Autodesk Fusion 360 part; units mm, degrees
note: some values were not read from the file. Set by a fixed rule: which sketch regions a step uses.
(part 2 of 3)
  arc A260 (-243, 45) -> (-241, 43) centre (-241, 45) ccw
  line L698 (-243, 45) -> (-243, 51)
  arc A261 (-243, 51) -> (-245, 53) centre (-245, 51) ccw
  line L699 (-245, 53) -> (-267, 53)
  line L700 (-267, 124) -> (-204, 124.0001)
  arc A262 (-204, 124.0001) -> (-202, 126.0001) centre (-204, 126.0001) ccw
  line L701 (-202, 126.0001) -> (-202, 135)
  line L702 (-202, 135) -> (-197, 135)
  line L703 (-197, 135) -> (-197, 133.0001)
  arc A263 (-197, 133.0001) -> (-195, 131.0001) centre (-195, 133.0001) ccw
  arc A264 (-172, 127) -> (-176, 131.0001) centre (-176, 127.0001) ccw
  line L704 (-172, 123) -> (-172, 127)
  arc A265 (-176, 119.0001) -> (-172, 123) centre (-176, 123.0001) ccw
  arc A266 (-195, 119) -> (-197, 117) centre (-195, 117) ccw
  line L705 (-197, 117) -> (-197, 115)
  line L706 (-197, 115) -> (-200, 115)
  arc A267 (-200, 115) -> (-202, 113) centre (-200, 113) ccw
  line L707 (-202, 109) -> (-202, 113)
  arc A268 (-204, 107) -> (-202, 109) centre (-204, 109) ccw
  line L708 (-204, 107) -> (-241, 107)
  arc A269 (-241, 107) -> (-243, 105) centre (-241, 105) ccw
  line L709 (-243, 105) -> (-243, 99)
  arc A270 (-245, 97) -> (-243, 99) centre (-245, 99) ccw
  line L710 (-245, 97) -> (-267, 97)
  arc A271 (-332, 126.0001) -> (-330, 124.0001) centre (-330, 126.0001) ccw
  line L711 (-332, 126.0001) -> (-332, 135)
  line L712 (-332, 135) -> (-337, 135)
  line L713 (-337, 135) -> (-337, 133.0001)
  arc A272 (-339, 131.0001) -> (-337, 133.0001) centre (-339, 133.0001) ccw
  arc A273 (-358, 131.0001) -> (-362, 127) centre (-358, 127.0001) ccw
  line L714 (-362, 123) -> (-362, 127)
  arc A274 (-362, 123) -> (-358, 119.0001) centre (-358, 123.0001) ccw
  arc A275 (-337, 117) -> (-339, 119) centre (-339, 117) ccw
  line L715 (-337, 117) -> (-337, 115)
  line L716 (-337, 115) -> (-334, 115)
  arc A276 (-332, 113) -> (-334, 115) centre (-334, 113) ccw
  line L717 (-332, 109) -> (-332, 113)
  arc A277 (-332, 109) -> (-330, 107) centre (-330, 109) ccw
  line L718 (-330, 107) -> (-287, 107)
  arc A278 (-285, 105) -> (-287, 107) centre (-287, 105) ccw
  line L719 (-285, 105) -> (-285, 99)
  arc A279 (-285, 99) -> (-283, 97) centre (-283, 99) ccw
  line L720 (-283, 97) -> (-267, 97)
  line L721 (-267, 124) -> (-330, 124.0001)
  line L722 (-327, 5) -> (-327, 10)
  line L723 (-327, 10) -> (-307, 10)
  arc A280 (-223, 3) -> (-225, 5) centre (-225, 3) ccw
  line L724 (-225, 5) -> (-227, 5)
  line L725 (-227, 5) -> (-227, 10)
  line L726 (-207, 10) -> (-227, 10)
  line L727 (-207, 5) -> (-207, 10)
  line L728 (-207, 5) -> (-209.0021, 5)
  arc A281 (-209.0021, 5) -> (-211.0021, 2.9998) centre (-209.0021, 3) ccw
  line L729 (-211, -15.9146) -> (-211.0021, 2.9998)
  arc A282 (-215, -19.9102) -> (-211, -15.9146) centre (-215, -15.9102) ccw
  line L730 (-219, -19.9102) -> (-215, -19.9102)
  arc A283 (-223, -15.9116) -> (-219, -19.9102) centre (-219, -15.9102) ccw
  line L731 (-223, -15.9116) -> (-223, 3)
  line L732 (-225, 145) -> (-227, 145)
  line L733 (-227, 145) -> (-227, 140)
  line L734 (-207, 140) -> (-227, 140)
  line L735 (-207, 145) -> (-207, 140)
  line L736 (-207, 145) -> (-209.0021, 145)
  arc A284 (-211.0021, 147.0002) -> (-209.0021, 145) centre (-209.0021, 147) ccw
  line L737 (-211.0007, 166.0733) -> (-211.0021, 147.0002)
  arc A285 (-211.0007, 166.0733) -> (-215, 170) centre (-215, 166) ccw
  line L738 (-219, 170) -> (-215, 170)
  arc A286 (-219, 170) -> (-223, 166.0009) centre (-219, 166) ccw
  line L739 (-223, 166.0009) -> (-223, 147)
  arc A287 (-225, 145) -> (-223, 147) centre (-225, 147) ccw
  arc A288 (-311, 147) -> (-309, 145) centre (-309, 147) ccw
  line L740 (-309, 145) -> (-307, 145)
  line L741 (-307, 145) -> (-307, 140)
  line L742 (-327, 140) -> (-307, 140)
  line L743 (-327, 145) -> (-327, 140)
  line L744 (-327, 145) -> (-324.9979, 145)
  arc A289 (-324.9979, 145) -> (-322.9979, 147.0002) centre (-324.9979, 147) ccw
  line L745 (-322.9993, 165.9261) -> (-322.9979, 147.0002)
  arc A290 (-319, 170) -> (-322.9993, 165.9261) centre (-319, 166) ccw
  line L746 (-315, 170) -> (-319, 170)
  arc A291 (-311, 166.0009) -> (-315, 170) centre (-315, 166) ccw
  line L747 (-311, 166.0009) -> (-311, 147)
  circle A292 centre (43.5, 122.75) radius 3
  circle A293 centre (58.5, 122.75) radius 3
  circle A294 centre (73.5, 122.75) radius 3
  circle A295 centre (73.5, 27.25) radius 3
  arc A296 (79.466, 30.6504) -> (82, 35) centre (77, 35) ccw
  circle A297 centre (43.5, 17.25) radius 2.5
  circle A298 centre (58.5, 17.25) radius 2.5
  circle A299 centre (73.5, 132.75) radius 2.5
  circle A300 centre (58.5, 132.75) radius 2.5
  circle A301 centre (43.5, 132.75) radius 2.5
  line L748 (35, 5) -> (35, 10)
  line L749 (57.5, 5) -> (35, 5)
  line L750 (57.5, 10) -> (35, 10)
  line L751 (57.5, 5) -> (80, 5)
  line L752 (80, 5) -> (80, 10)
  line L753 (80, 10) -> (57.5, 10)
  line L754 (-10, -124) -> (-10, -114)
  line L755 (-10, -59) -> (-10, -69)
  line L756 (-13, -74) -> (-12, -74)
  line L757 (-12, -109) -> (-13, -109)
  line L758 (-15, -117) -> (-15, -114)
  arc A302 (-13, -109) -> (-14.3301, -109.5064) centre (-13, -111) ccw
  arc A303 (-12, -109) -> (-10, -107) centre (-12, -107) ccw
  arc A304 (-10, -76) -> (-12, -74) centre (-12, -76) ccw
  line L759 (-10, -76) -> (-10, -80.6987)
  line L760 (-10, -88.0192) -> (-10, -98.0192)
  arc A305 (-15, -72) -> (-14.9997, -72.0383) centre (-13, -72) ccw
  arc A306 (-14.3301, -73.4936) -> (-13, -74) centre (-13, -72) ccw
  line L761 (-15, -72) -> (-15, -67)
  line L762 (-135.6699, -107.8397) -> (-140, -105.3397)
  line L763 (-135.6699, -109.5064) -> (-135.6699, -107.8397)
  arc A307 (-135.6699, -109.5064) -> (-137, -109) centre (-137, -111) ccw
  line L764 (-138, -109) -> (-137, -109)
  line L765 (-140, -105.3398) -> (-140, -107)
  arc A308 (-140, -107) -> (-138, -109) centre (-138, -107) ccw
  line L766 (-139.9897, -75.7973) -> (-140, -80.6987)
  line L767 (-140, -80.6987) -> (-135.6699, -78.1987)
  arc A309 (-137, -74) -> (-135.6699, -73.4936) centre (-137, -72) ccw
  line L768 (-137, -74) -> (-138, -74)
  arc A310 (-138, -74) -> (-140, -76) centre (-138, -76) ccw
  line L769 (-140, -76) -> (-140, -80.6987)
  line L770 (-135.6699, -78.1987) -> (-135.6699, -73.4936)
  arc A311 (-133, -64) -> (-135, -66) centre (-133, -66) ccw
  line L771 (-133, -64) -> (-132, -64)
  arc A312 (-132, -64) -> (-131.6546, -63.9699) centre (-132, -62) ccw
  line L772 (-130.6699, -64.5385) -> (-131.6546, -63.9699)
  line L773 (-130.6699, -69.5385) -> (-130.6699, -64.5385)
  line L774 (-135, -72.0385) -> (-130.6699, -69.5385)
  line L775 (-135.0004, -72.0383) -> (-135, -72.0385)
  arc A313 (-135.0004, -72.0383) -> (-135, -72) centre (-137, -72) ccw
  line L776 (-135, -67) -> (-135, -66)
  line L777 (-135, -72) -> (-135, -67)
  line L778 (-90, -124) -> (-90, -129)
  line L779 (-90, -124) -> (-115, -124)
  line L780 (-115, -124) -> (-115, -129)
  line L781 (-115, -129) -> (-135, -129)
  line L782 (-135, -124) -> (-140, -124)
  line L783 (-140, -124) -> (-140, -114)
  line L784 (-145, -114) -> (-140, -114)
  line L785 (-145, -69) -> (-145, -114)
  line L786 (-140, -69) -> (-145, -69)
  line L787 (-140, -59) -> (-140, -69)
  line L788 (-140, -59) -> (-135, -59)
  line L789 (-135, -54) -> (-135, -59)
  line L790 (-135, -49) -> (-135, -54)
  arc A314 (-131.8566, -44.3575) -> (-135, -49) centre (-130, -49) ccw
  arc A315 (-115, -49) -> (-118.1434, -44.3575) centre (-120, -49) ccw
  line L791 (-115, -54) -> (-115, -49)
  line L792 (-115, -59) -> (-115, -54)
  line L793 (-115, -59) -> (-94.5, -59)
  line L794 (-94.5, -59) -> (-94.5, -39)
  arc A316 (-89.5, -34) -> (-94.5, -39) centre (-89.5, -39) ccw
  line L795 (-135, -129) -> (-135, -124)
  line L796 (-90, -129) -> (-60, -129)
  circle A317 centre (-85, -48) radius 4.075
  circle A318 centre (-371, 85) radius 4.075
  line L797 (-438, 19) -> (-442, 19)
  line L798 (-444, 17) -> (-444, 15.5)
  line L799 (-442, 13.5) -> (-438, 13.5)
  line L800 (-436, 15.5) -> (-436, 17)
  arc A319 (-436, 17) -> (-438, 19) centre (-438, 17) ccw
  arc A320 (-438, 13.5) -> (-436, 15.5) centre (-438, 15.5) ccw
  arc A321 (-444, 15.5) -> (-442, 13.5) centre (-442, 15.5) ccw
  arc A322 (-442, 19) -> (-444, 17) centre (-442, 17) ccw
  arc A323 (-438, 131) -> (-436, 133) centre (-438, 133) ccw
  line L801 (-438, 131) -> (-442, 131)
  arc A324 (-444, 133) -> (-442, 131) centre (-442, 133) ccw
  line L802 (-444, 133) -> (-444, 134.5)
  arc A325 (-442, 136.5) -> (-444, 134.5) centre (-442, 134.5) ccw
  line L803 (-442, 136.5) -> (-438, 136.5)
  arc A326 (-436, 134.5) -> (-438, 136.5) centre (-438, 134.5) ccw
  line L804 (-436, 134.5) -> (-436, 133)
  arc A327 (41.7475, 118.6053) -> (45.2525, 118.6053) centre (43.5, 122.75) ccw
  line L805 (34, 119) -> (39.8003, 119)
  line L806 (47.1997, 119) -> (54.8003, 119)
  arc A328 (56.7475, 118.6053) -> (60.2525, 118.6053) centre (58.5, 122.75) ccw
  line L807 (62.1997, 119) -> (69.8003, 119)
  line L808 (77.1997, 119) -> (81, 119)
  arc A329 (71.7475, 118.6053) -> (75.2525, 118.6053) centre (73.5, 122.75) ccw
  arc A330 (41.7475, 118.6053) -> (39.8003, 119) centre (39.8003, 114) ccw
  arc A331 (47.1997, 119) -> (45.2525, 118.6053) centre (47.1997, 114) ccw
  arc A332 (56.7475, 118.6053) -> (54.8003, 119) centre (54.8003, 114) ccw
  arc A333 (62.1997, 119) -> (60.2525, 118.6053) centre (62.1997, 114) ccw
  arc A334 (71.7475, 118.6053) -> (69.8003, 119) centre (69.8003, 114) ccw
  arc A335 (77.1997, 119) -> (75.2525, 118.6053) centre (77.1997, 114) ccw
  line L809 (-82.0096, -106.5) -> (-77.9904, -106.5)
  line L810 (-72.0096, -106.5) -> (-67.9904, -106.5)
  arc A336 (-289.5, 21) -> (-291.5, 23) centre (-291.5, 21) ccw
  line L811 (-291.5, 23) -> (-327, 23)
  arc A337 (-327, 23) -> (-329, 21) centre (-327, 21) ccw
  line L812 (-329, 15) -> (-329, 21)
  arc A338 (-329, 15) -> (-327, 13) centre (-327, 15) ccw
  line L813 (-249.5, 23) -> (-284.5, 23)
  arc A339 (-284.5, 23) -> (-286.5, 21) centre (-284.5, 21) ccw
  arc A340 (-247.5, 21) -> (-249.5, 23) centre (-249.5, 21) ccw
  line L814 (-337, 108) -> (-337, 92.5)
  arc A341 (-337, 108) -> (-339, 110) centre (-339, 108) ccw
  line L815 (-339, 110) -> (-340, 110)
  arc A342 (-342, 112) -> (-340, 110) centre (-340, 112) ccw
  line L816 (-342, 112) -> (-342, 112.9999)
  arc A343 (-342, 112.9999) -> (-344, 114.9999) centre (-344, 112.9999) ccw
  arc A344 (-366, 122.9999) -> (-358, 114.9999) centre (-358, 122.9999) ccw
  line L817 (-366, 126.9998) -> (-366, 122.9999)
  arc A345 (-358, 134.9998) -> (-366, 126.9998) centre (-358, 126.9998) ccw
  arc A346 (-344, 134.9999) -> (-342, 136.9999) centre (-344, 136.9999) ccw
  line L818 (-342, 136.9999) -> (-342.0001, 145)
  arc A347 (-337, 150) -> (-342.0001, 145) centre (-337, 145) ccw
  line L819 (-337, 150) -> (-329, 150)
  arc A348 (-329, 150) -> (-327, 152) centre (-329, 152) ccw
  line L820 (-327, 166) -> (-327, 152)
  arc A349 (-319, 174) -> (-327, 166) centre (-319, 166) ccw
  line L821 (-315, 174) -> (-319, 174)
  arc A350 (-307, 166.0013) -> (-315, 174) centre (-315, 166) ccw
  line L822 (-307, 152) -> (-307, 166.0013)
  arc A351 (-307, 152) -> (-305, 150) centre (-305, 152) ccw
  line L823 (-305, 150) -> (-304, 150)
  arc A352 (-302, 148) -> (-304, 150) centre (-304, 148) ccw
  line L824 (-302, 147) -> (-302, 148)
  arc A353 (-302, 147) -> (-300, 145) centre (-300, 147) ccw
  line L825 (-300, 145) -> (-286.5, 145)
  line L826 (-247.5, 144.9999) -> (-233.9999, 144.9999)
  arc A354 (-233.9999, 144.9999) -> (-231.9997, 147.0001) centre (-233.9999, 147.0001) ccw
  line L827 (-231.9997, 147.0001) -> (-231.9997, 147.9994)
  arc A355 (-229.999, 150.0001) -> (-231.9997, 147.9994) centre (-229.999, 147.9994) ccw
  line L828 (-229, 150.0001) -> (-229.999, 150.0001)
  arc A356 (-229, 150.0001) -> (-227, 152.0001) centre (-229, 152.0001) ccw
  line L829 (-227, 152.0001) -> (-227, 166.002)
  arc A357 (-219, 174) -> (-227, 166.002) centre (-219, 166) ccw
  line L830 (-219, 174) -> (-215, 174)
  arc A358 (-207, 166) -> (-215, 174) centre (-215, 166) ccw
  line L831 (-207, 166) -> (-207, 152.0001)
  arc A359 (-207, 152.0001) -> (-205, 150.0001) centre (-205, 152.0001) ccw
  line L832 (-197, 150.0001) -> (-205, 150.0001)
  arc A360 (-192, 145.0001) -> (-197, 150.0001) centre (-197, 145.0001) ccw
  line L833 (-192, 145.0001) -> (-192, 136.9999)
  arc A361 (-192, 136.9999) -> (-190, 134.9999) centre (-190, 136.9999) ccw
  arc A362 (-168, 126.9998) -> (-175.9914, 134.9998) centre (-176, 126.9998) ccw
  line L834 (-168, 126.9998) -> (-168, 122.9999)
  arc A363 (-176, 114.9999) -> (-168, 122.9999) centre (-176, 122.9999) ccw
  arc A364 (-190, 114.9999) -> (-192, 112.9999) centre (-190, 112.9999) ccw
  line L835 (-192, 112) -> (-192, 112.9999)
  arc A365 (-194, 110) -> (-192, 112) centre (-194, 112) ccw
  line L836 (-195, 110) -> (-194, 110)
  arc A366 (-195, 110) -> (-197, 108) centre (-195, 108) ccw
  line L837 (-197, 108) -> (-197, 90)
  line L838 (-197, 90) -> (-202, 90)
  line L839 (-202, 90) -> (-202, 75)
  arc A367 (-406.5714, 84.2084) -> (-403.2084, 87.5714) centre (-408, 89) ccw
  arc A368 (-401.2918, 89) -> (-403.2084, 87.5714) centre (-401.2918, 87) ccw
  arc A369 (-386.7082, 61) -> (-384.7916, 62.4286) centre (-386.7082, 63) ccw
  arc A370 (-381.4286, 65.7916) -> (-384.7916, 62.4286) centre (-380, 61) ccw
  arc A371 (-381.4286, 65.7916) -> (-380, 67.7082) centre (-382, 67.7082) ccw
  arc A372 (-406.5714, 84.2084) -> (-408, 82.2918) centre (-406, 82.2918) ccw
  circle A373 centre (-408, 89) radius 1
  circle A374 centre (-380, 61) radius 1
  line L840 (-408, 82.2918) -> (-408, 67.7082)
  line L841 (-401.2918, 61) -> (-386.7082, 61)
  line L842 (-401.2918, 89) -> (-386.7082, 89)
  line L843 (-380, 82.2918) -> (-380, 67.7082)
  line L844 (-104, 5) -> (-86, 5)
  line L845 (-56, 5) -> (-38, 5)
  line L846 (-104, 145) -> (-86, 145)
  line L847 (-56, 145) -> (-38, 145)
  line L848 (-141, 90) -> (-141, 108)
  line L849 (-141, 60) -> (-141, 42)
  line L850 (-302, 8) -> (-291.5, 8)
  line L851 (-327, 13) -> (-306, 13)
  line L852 (-304, 11) -> (-304, 10)
  line L853 (-289.5, 21) -> (-289.5, 10)
  arc A375 (-304, 11) -> (-306, 13) centre (-306, 11) ccw
  arc A376 (-304, 10) -> (-302, 8) centre (-302, 10) ccw
  arc A377 (-291.5, 8) -> (-289.5, 10) centre (-291.5, 10) ccw
  arc A378 (-244.5001, 10) -> (-242.5001, 8) centre (-242.5001, 10) ccw
  line L854 (-232.0001, 7.9999) -> (-242.5001, 8)
  arc A379 (-232.0001, 7.9999) -> (-230.0001, 9.9999) centre (-232.0001, 9.9999) ccw
  line L855 (-230.0001, 10.9999) -> (-230.0001, 9.9999)
  arc A380 (-228.0001, 12.9999) -> (-230.0001, 10.9999) centre (-228.0001, 10.9999) ccw
  line L856 (-207.0001, 12.9999) -> (-228.0001, 12.9999)
  arc A381 (-207.0001, 12.9999) -> (-205.0001, 14.9999) centre (-207.0001, 14.9999) ccw
  line L857 (-205.0001, 14.9999) -> (-205.0001, 20.9999)
  arc A382 (-205.0001, 20.9999) -> (-207.0001, 22.9999) centre (-207.0001, 20.9999) ccw
  line L858 (-242.4962, 23) -> (-207.0001, 22.9999)
  arc A383 (-242.4962, 23) -> (-244.5001, 21) centre (-242.5001, 21) ccw
  line L859 (-244.5001, 21) -> (-244.5001, 10)
  line L860 (-329, 135) -> (-329, 129)
  arc A384 (-327, 137) -> (-329, 135) centre (-327, 135) ccw
  line L861 (-327, 137) -> (-306, 137)
  arc A385 (-306, 137) -> (-304, 139) centre (-306, 139) ccw
  line L862 (-304, 139) -> (-304, 140)
  arc A386 (-302, 142) -> (-304, 140) centre (-302, 140) ccw
  line L863 (-302, 142) -> (-291.5, 142)
  arc A387 (-289.5, 140) -> (-291.5, 142) centre (-291.5, 140) ccw
  line L864 (-289.5, 129) -> (-289.5, 140)
  arc A388 (-291.5, 127) -> (-289.5, 129) centre (-291.5, 129) ccw
  line L865 (-291.5, 127) -> (-327, 127)
  arc A389 (-329, 129) -> (-327, 127) centre (-327, 129) ccw
  arc A390 (-207.0001, 127.0001) -> (-205.0001, 129.0001) centre (-207.0001, 129.0001) ccw
  line L866 (-205.0001, 135.0001) -> (-205.0001, 129.0001)
  arc A391 (-205.0001, 135.0001) -> (-207.0001, 137.0001) centre (-207.0001, 135.0001) ccw
  line L867 (-207.0001, 137.0001) -> (-228.0001, 137.0001)
  arc A392 (-230.0001, 139.0001) -> (-228.0001, 137.0001) centre (-228.0001, 139.0001) ccw
  line L868 (-230.0001, 139.0001) -> (-230.0001, 140.0001)
  arc A393 (-230.0001, 140.0001) -> (-232.0001, 142.0001) centre (-232.0001, 140.0001) ccw
  line L869 (-232.0001, 142.0001) -> (-242.5001, 142)
  arc A394 (-242.5001, 142) -> (-244.5001, 140) centre (-242.5001, 140) ccw
  line L870 (-244.5001, 129) -> (-244.5001, 140)
  arc A395 (-244.5001, 129) -> (-242.4962, 127) centre (-242.5001, 129) ccw
  line L871 (-242.4962, 127) -> (-207.0001, 127.0001)
  line L872 (-437, 10) -> (-392, 10)
  line L873 (-414.5, 145) -> (-392, 145)
  line L874 (-414.5, 145) -> (-437, 145)
  line L875 (-437, 145) -> (-437, 140)
  line L876 (-437, 140) -> (-392, 140)
  line L877 (-392, 145) -> (-392, 140)
  line L878 (-418.1847, 13) -> (-405.8153, 13)
  arc A396 (-422.7659, 14.1111) -> (-418.1847, 13) centre (-418.1847, 23) ccw
  arc A397 (-405.8153, 13) -> (-401.2341, 14.1111) centre (-405.8153, 23) ccw
  line L879 (-136, 10) -> (-141, 10)
  line L880 (-141, 5) -> (-136, 5)
  line L881 (-136, 5) -> (-136, 10)
  line L882 (-141, 10) -> (-141, 5)
  line L883 (-1, 5) -> (-6, 5)
  line L884 (-6, 5) -> (-6, 10)
  line L885 (-6, 10) -> (-1, 10)
  line L886 (-1, 10) -> (-1, 5)
  line L887 (-136, 145) -> (-136, 140)
  line L888 (-136, 140) -> (-141, 140)
  line L889 (-141, 140) -> (-141, 145)
  line L890 (-141, 145) -> (-136, 145)
  line L891 (-6, 145) -> (-6, 140)
  line L892 (-6, 140) -> (-1, 140)
  line L893 (-1, 140) -> (-1, 145)
  line L894 (-1, 145) -> (-6, 145)
  arc A398 (-403.2084, 62.4286) -> (-406.5714, 65.7916) centre (-408, 61) ccw
  arc A399 (-411.2142, 57.17) -> (-406.0857, 56.381) centre (-408, 61) ccw
  arc A400 (-401.2341, 14.1111) -> (-402.0555, 56.2922) centre (-412, 35) ccw
  arc A401 (-415.0846, 58.2967) -> (-422.7659, 14.1111) centre (-412, 35) ccw
  arc A402 (-411.2142, 57.17) -> (-415.0846, 58.2967) centre (-414.4283, 53.3399) ccw
  arc A403 (-402.0555, 56.2922) -> (-406.0857, 56.381) centre (-404.1714, 51.7619) ccw
  line L895 (-418.1847, 137) -> (-405.8153, 137)
  arc A404 (-401.2341, 135.8889) -> (-405.8153, 137) centre (-405.8153, 127) ccw
  arc A405 (-402.0555, 93.7078) -> (-401.2341, 135.8889) centre (-412, 115) ccw
  arc A406 (-406.0857, 93.619) -> (-402.0555, 93.7078) centre (-404.1714, 98.2381) ccw
  arc A407 (-406.0857, 93.619) -> (-411.2142, 92.83) centre (-408, 89) ccw
  arc A408 (-415.0846, 91.7033) -> (-411.2142, 92.83) centre (-414.4283, 96.6601) ccw
  arc A409 (-422.7659, 135.8889) -> (-415.0846, 91.7033) centre (-412, 115) ccw
  arc A410 (-418.1847, 137) -> (-422.7659, 135.8889) centre (-418.1847, 127) ccw
  circle A411 centre (-125, -40) radius 2.5
  arc A412 (-119.3006, -41.8753) -> (-130.6994, -41.8753) centre (-125, -40) ccw
  arc A413 (-119.3006, -41.8753) -> (-118.1434, -44.3575) centre (-117.4008, -42.5004) ccw
  arc A414 (-131.8566, -44.3575) -> (-130.6994, -41.8753) centre (-132.5992, -42.5004) ccw
  arc A415 (-15, -49) -> (-18.1435, -44.3575) centre (-20, -49) ccw
  arc A416 (-19.3006, -41.8753) -> (-18.1435, -44.3575) centre (-17.4008, -42.5004) ccw
  arc A417 (-19.3006, -41.8753) -> (-30.6994, -41.8753) centre (-25, -40) ccw
  circle A418 centre (-25, -40) radius 2.5
  arc A419 (-31.8566, -44.3575) -> (-35, -49) centre (-30, -49) ccw
  arc A420 (-31.8566, -44.3575) -> (-30.6994, -41.8753) centre (-32.5992, -42.5004) ccw
  line L896 (-286.5, 5) -> (-286.5, 11)
  line L897 (-284.5, 13) -> (-249.5, 13)
  line L898 (-247.5, 11) -> (-247.5, 5.0001)
  arc A421 (-249.5, 16) -> (-247.5, 18) centre (-249.5, 18) ccw
  line L899 (-249.5, 16) -> (-284.5, 16)
  arc A422 (-286.5, 18) -> (-284.5, 16) centre (-284.5, 18) ccw
  arc A423 (-284.5, 13) -> (-286.5, 11) centre (-284.5, 11) ccw
  arc A424 (-247.5, 11) -> (-249.5, 13) centre (-249.5, 11) ccw
  line L900 (-286.5, 18) -> (-286.5, 21)
  line L901 (-247.5, 21) -> (-247.5, 18)
  line L902 (-284.5, 137) -> (-249.5, 137)
  arc A425 (-284.5, 134) -> (-286.5, 132) centre (-284.5, 132) ccw
  line L903 (-286.5, 132) -> (-286.5, 129)
  arc A426 (-286.5, 129) -> (-284.5, 127) centre (-284.5, 129) ccw
  line L904 (-249.5, 127) -> (-284.5, 127)
  arc A427 (-249.5, 127) -> (-247.5, 129) centre (-249.5, 129) ccw
  line L905 (-247.5, 129) -> (-247.5, 132)
  arc A428 (-247.5, 132) -> (-249.5, 134) centre (-249.5, 132) ccw
  line L906 (-249.5, 134) -> (-284.5, 134)
  arc A429 (-286.5, 139) -> (-284.5, 137) centre (-284.5, 139) ccw
  line L907 (-286.5, 145) -> (-286.5, 139)
  line L908 (-247.5, 139) -> (-247.5, 144.9999)
  arc A430 (-249.5, 137) -> (-247.5, 139) centre (-249.5, 139) ccw
  line L909 (-337, 92.5) -> (-331, 92.5)
  line L910 (-337, 57.5) -> (-331, 57.5)
  line L911 (-329, 90.5) -> (-329, 59.5)
  arc A431 (-329, 90.5) -> (-331, 92.5) centre (-331, 90.5) ccw
  arc A432 (-331, 57.5) -> (-329, 59.5) centre (-331, 59.5) ccw
  arc A433 (76.1918, 30.8561) -> (70.8974, 30.9211) centre (73.5, 27.25) ccw
  line L912 (38, 30) -> (68.0057, 30)
  arc A434 (68.0057, 30) -> (70.8974, 30.9211) centre (68.0057, 35) ccw
  arc A435 (76.1918, 30.8561) -> (79.466, 30.6504) centre (77.9864, 33.2602) ccw
  line L913 (-195, 18.9999) -> (-176, 18.9999)
  line L914 (-190, 15.0001) -> (-175.9914, 15.0002)
  line L915 (-190, 35.0001) -> (-176, 35.0001)
  line L916 (-195, 31) -> (-176, 30.9999)
  line L917 (-195, 119) -> (-176, 119.0001)
  line L918 (-190, 114.9999) -> (-176, 114.9999)
  line L919 (-195, 131.0001) -> (-176, 131.0001)
  line L920 (-190, 134.9999) -> (-175.9914, 134.9998)
  line L921 (-358, 134.9998) -> (-344, 134.9999)
  line L922 (-358, 131.0001) -> (-339, 131.0001)
  line L923 (-358, 119.0001) -> (-339, 119)
  line L924 (-358, 114.9999) -> (-344, 114.9999)
  line L925 (-358, 35.0001) -> (-344, 35.0001)
  line L926 (-358, 30.9999) -> (-339, 31)
  line L927 (-358, 18.9999) -> (-339, 18.9999)
  line L928 (-358, 15.0002) -> (-344, 15.0001)
  circle A436 centre (-240, 91) radius 1.5
  circle A437 centre (-208, 91) radius 1.5
  circle A438 centre (-240, 59) radius 1.5
  circle A439 centre (-208, 59) radius 1.5
  line L929 (-240, 65.3246) -> (-240, 84.6754)
  line L930 (-214.3246, 59) -> (-233.6754, 59)
  line L931 (-238.5, 59) -> (-240, 59)
  arc A440 (-236.386, 60.7143) -> (-238.2857, 62.614) centre (-240, 59) ccw
  arc A441 (-238.2857, 87.386) -> (-236.386, 89.2857) centre (-240, 91) ccw
  arc A442 (-211.614, 89.2857) -> (-209.7143, 87.386) centre (-208, 91) ccw
  line L932 (-233.6754, 91) -> (-214.3246, 91)
  line L933 (-208, 84.6754) -> (-208, 65.3246)
  arc A443 (-209.7143, 62.614) -> (-211.614, 60.7143) centre (-208, 59) ccw
  arc A444 (-238.2857, 87.386) -> (-240, 84.6754) centre (-237, 84.6754) ccw
  arc A445 (-233.6754, 91) -> (-236.386, 89.2857) centre (-233.6754, 88) ccw
  arc A446 (-240, 65.3246) -> (-238.2857, 62.614) centre (-237, 65.3246) ccw
  arc A447 (-236.386, 60.7143) -> (-233.6754, 59) centre (-233.6754, 62) ccw
  arc A448 (-214.3246, 59) -> (-211.614, 60.7143) centre (-214.3246, 62) ccw
  arc A449 (-209.7143, 62.614) -> (-208, 65.3246) centre (-211, 65.3246) ccw
  arc A450 (-208, 84.6754) -> (-209.7143, 87.386) centre (-211, 84.6754) ccw
  arc A451 (-211.614, 89.2857) -> (-214.3246, 91) centre (-214.3246, 88) ccw
  circle A452 centre (30, -80) radius 1
  circle A453 centre (30, -108) radius 1
  arc A454 (31.1111, -82.2395) -> (32.2395, -81.1111) centre (30, -80) ccw
  line L934 (30, -103.9689) -> (30, -84.0311)
  line L935 (34.0311, -80) -> (44, -80)
  arc A455 (30, -103.9689) -> (31.1111, -105.7605) centre (32, -103.9689) ccw
  arc A456 (34.0311, -80) -> (32.2395, -81.1111) centre (34.0311, -82) ccw
  arc A457 (31.1111, -82.2395) -> (30, -84.0311) centre (32, -84.0311) ccw
  line L936 (19.75, -89.25) -> (19.75, -95.75)
  line L937 (22.25, -89.2502) -> (22.25, -95.75)
  arc A458 (22.25, -89.2502) -> (19.75, -89.25) centre (21, -89.25) ccw
  arc A459 (19.75, -95.75) -> (22.25, -95.75) centre (21, -95.75) ccw
  line L938 (-75, -55) -> (-90, -55)
  line L939 (-92, -57) -> (-92, -103)
  line L940 (-90, -105) -> (-60, -105)
  line L941 (-58, -103) -> (-58, -57)
  line L942 (-60, -55) -> (-75, -55)
  arc A460 (22.25, -107.25) -> (19.75, -107.25) centre (21, -107.25) ccw
  line L943 (19.75, -113.75) -> (19.75, -107.25)
  arc A461 (19.75, -113.75) -> (22.25, -113.7498) centre (21, -113.75) ccw
  line L944 (22.25, -113.7498) -> (22.25, -107.25)
  line L945 (-87.9002, -106.5521) -> (-92.1651, -106.5898)
  line L946 (-62.0096, -106.5) -> (-57.9904, -106.5)
  arc A462 (-90, -55) -> (-92, -57) centre (-90, -57) ccw
  arc A463 (-58, -57) -> (-60, -55) centre (-60, -57) ccw
  arc A464 (-60, -105) -> (-58, -103) centre (-60, -103) ccw
  arc A465 (-92, -103) -> (-90, -105) centre (-90, -103) ccw
  line L947 (-89.5, -34) -> (-60.5, -34)
  arc A466 (32.5, -108) -> (31.1111, -105.7605) centre (30, -108) ccw
  line L948 (21, -99.7811) -> (21, -103.2189)
  line L949 (32.5, -108) -> (32.5, -110.7498)
  line L950 (29.5, -113.7498) -> (25.0312, -113.7498)
  line L951 (18.5, -113.7498) -> (18.5, -107.25)
  line L952 (18.5, -95.75) -> (18.5, -89.25)
  arc A467 (18.5, -113.7498) -> (23.2396, -114.861) centre (21, -113.75) ccw
  arc A468 (19.8889, -105.0105) -> (18.5, -107.25) centre (21, -107.25) ccw
  arc A469 (18.5, -95.75) -> (19.8889, -97.9895) centre (21, -95.75) ccw
  line L953 (30, -77.5) -> (44, -77.5)
  arc A470 (31.1111, -82.2395) -> (32.2395, -81.1111) centre (30, -80) ccw
  arc A471 (30, -77.5) -> (27.5, -80) centre (30, -80) ccw
  arc A472 (21, -99.7811) -> (19.8889, -97.9895) centre (19, -99.7811) ccw
  arc A473 (19.8889, -105.0105) -> (21, -103.2189) centre (19, -103.2189) ccw
  arc A474 (25.0312, -113.7498) -> (23.2396, -114.861) centre (25.0312, -115.7498) ccw
  arc A475 (29.5, -113.7498) -> (32.5, -110.7498) centre (29.5, -110.7498) ccw
  circle A476 centre (58, -108) radius 1
  line L954 (68.25, -113.75) -> (68.25, -107.25)
  arc A477 (65.75, -113.7498) -> (68.25, -113.75) centre (67, -113.75) ccw
  arc A478 (68.25, -107.25) -> (65.75, -107.25) centre (67, -107.25) ccw
  line L955 (65.75, -113.7498) -> (65.75, -107.25)
  arc A479 (65.75, -95.75) -> (68.25, -95.75) centre (67, -95.75) ccw
  line L956 (68.25, -89.25) -> (68.25, -95.75)
  arc A480 (68.25, -89.25) -> (65.75, -89.2502) centre (67, -89.25) ccw
  line L957 (65.75, -89.2502) -> (65.75, -95.75)
  circle A481 centre (58, -80) radius 1
  line L958 (-55.25, -93.75) -> (-48.75, -93.75)
  line L959 (-55.25, -96.25) -> (-48.75, -96.25)
  arc A482 (-55.25, -93.75) -> (-55.25, -96.25) centre (-55.25, -95) ccw
  arc A483 (-48.75, -96.25) -> (-48.75, -93.75) centre (-48.75, -95) ccw
  line L960 (-55.25, -75.75) -> (-48.75, -75.75)
  arc A484 (-55.25, -75.75) -> (-55.25, -78.25) centre (-55.25, -77) ccw
  line L961 (-55.25, -78.25) -> (-48.75, -78.25)
  arc A485 (-48.75, -78.25) -> (-48.75, -75.75) centre (-48.75, -77) ccw
  line L962 (-94.75, -93.75) -> (-101.25, -93.75)
  arc A486 (-94.75, -96.25) -> (-94.75, -93.75) centre (-94.75, -95) ccw
  line L963 (-94.75, -96.25) -> (-101.25, -96.25)
  arc A487 (-101.25, -93.75) -> (-101.25, -96.25) centre (-101.25, -95) ccw
  line L964 (-94.75, -75.75) -> (-101.25, -75.75)
  arc A488 (-94.75, -78.25) -> (-94.75, -75.75) centre (-94.75, -77) ccw
  arc A489 (-101.25, -75.75) -> (-101.25, -78.25) centre (-101.25, -77) ccw
  line L965 (-94.75, -78.25) -> (-101.25, -78.25)
  line L966 (27.5, -80) -> (27.5, -87)
  line L967 (25.5, -89) -> (24.8971, -89)
  arc A490 (23.1651, -88) -> (18.5, -89.25) centre (21, -89.25) ccw
  arc A491 (23.1651, -88) -> (24.8971, -89) centre (24.8971, -87) ccw
  arc A492 (25.5, -89) -> (27.5, -87) centre (25.5, -87) ccw
  arc A493 (58, -84.0311) -> (56.8889, -82.2395) centre (56, -84.0311) ccw
  line L968 (58, -103.9689) -> (58, -84.0311)
  arc A494 (56.8889, -105.7605) -> (58, -103.9689) centre (56, -103.9689) ccw
  arc A495 (56.8889, -105.7605) -> (55.5, -108) centre (58, -108) ccw
  line L969 (55.5, -108) -> (55.5, -110.7498)
  arc A496 (55.5, -110.7498) -> (58.5, -113.7498) centre (58.5, -110.7498) ccw
  line L970 (58.5, -113.7498) -> (62.9688, -113.7498)
  arc A497 (64.7604, -114.861) -> (62.9688, -113.7498) centre (62.9688, -115.7498) ccw
  arc A498 (64.7604, -114.861) -> (69.5, -113.7498) centre (67, -113.75) ccw
  line L971 (69.5, -113.7498) -> (69.5, -107.25)
  arc A499 (69.5, -107.25) -> (68.1111, -105.0105) centre (67, -107.25) ccw
  arc A500 (67, -103.2189) -> (68.1111, -105.0105) centre (69, -103.2189) ccw
  line L972 (67, -99.7811) -> (67, -103.2189)
  arc A501 (68.1111, -97.9895) -> (67, -99.7811) centre (69, -99.7811) ccw
  arc A502 (68.1111, -97.9895) -> (69.5, -95.75) centre (67, -95.75) ccw
  line L973 (69.5, -95.75) -> (69.5, -89.25)
  arc A503 (69.5, -89.25) -> (64.8349, -88) centre (67, -89.25) ccw
  arc A504 (63.1029, -89) -> (64.8349, -88) centre (63.1029, -87) ccw
  line L974 (62.5, -89) -> (63.1029, -89)
  arc A505 (60.5, -87) -> (62.5, -89) centre (62.5, -87) ccw
  line L975 (60.5, -80) -> (60.5, -87)
  arc A506 (60.5, -80) -> (58, -77.5) centre (58, -80) ccw
  line L976 (58, -77.5) -> (44, -77.5)
  arc A507 (55.7605, -81.1111) -> (56.8889, -82.2395) centre (58, -80) ccw
  arc A508 (55.7605, -81.1111) -> (53.9689, -80) centre (53.9689, -82) ccw
  line L977 (53.9689, -80) -> (44, -80)
  point P0 (-192, 0)
  point P1 (-75, -119)
  point P2 (-80, -110.3397)
  point P3 (-120, -58.3782)
  point P4 (-75, -119)
  point P5 (-75.0001, -119)
  point P6 (-75, -119)
  point P7 (-75, -119)
  point P8 (-75, -119)
  point P9 (-70, -110.3397)
  point P10 (-75, -119)
  point P11 (-75, -119)
  point P12 (-30, -58.3782)
  point P13 (35, -40)
  point P14 (35, -35)
  point P15 (-92, -55)
  point P16 (-92, -105)
  point P17 (-58, -105)
  point P18 (44, -92.3923)
  dimension "d35" = 5
  dimension "d36" = 5
  dimension "d40" = 5
  dimension "d41" = 2
  dimension "d67" = 5
  dimension "d68" = 5
  dimension "d69" = 2
  dimension "d89" = 5
  dimension "d94" = 5
  dimension "d112" = 2.5
  dimension "d113" = 2.5
  dimension "d116" = 2.5
  dimension "d369" = 2
  dimension "d426" = 3
  dimension "d427" = 3
  dimension "d429" = 3
  dimension "d466" = 8
  dimension "d474" = 3
  dimension "d508" = 3
  dimension "d524" = 8
  dimension "d525" = 8
  dimension "d526" = 4
  dimension "d527" = 2
  dimension "d528" = 1
  dimension "d529" = 2
  dimension "d532" = 14
  dimension "d533" = 14
  dimension "d534" = 14
  dimension "d535" = 14
  dimension "d545" = 2
  dimension "d546" = 8
  dimension "d555" = 3
  dimension "d557" = 1
  dimension "d575" = 1
  dimension "d576" = 1
  dimension "d577" = 1
  dimension "d578" = 1
  dimension "d579" = 1
  dimension "d589" = 10
  dimension "d591" = 5
  dimension "d592" = 5
  dimension "d593" = 5
  dimension "d594" = 5
  dimension "d604" = 5
  dimension "d605" = 2
  dimension "d625" = 2
  dimension "d629" = 2
  dimension "d643" = 1
  dimension "d648" = 2
  dimension "d649" = 4
  dimension "d652" = 2
  dimension "d654" = 5
  dimension "d655" = 5
  dimension "d675" = 4
  dimension "d686" = 2
  dimension "d687" = 2
  dimension "d688" = 5
  dimension "d693" = 6
  dimension "d694" = 6
  dimension "d695" = 6
  dimension "d701" = 6
  dimension "d703" = 5
  dimension "d704" = 5
  dimension "d705" = 5
  dimension "d706" = 5
  dimension "d707" = 5
  dimension "d709" = 2
  dimension "d718" = 8.15
  dimension "d719" = 8.15
  dimension "d722" = 2
  dimension "d726" = 9
  dimension "d727" = 9
  dimension "d728" = 9
  dimension "d729" = 5
  dimension "d742" = 2
  dimension "d750" = 10
  dimension "d772" = 5
  dimension "d773" = 2
  dimension "d774" = 2
  dimension "d861" = 3
  dimension "d862" = 3
  dimension "d863" = 3
  dimension "d864" = 3
  dimension "d865" = 3
  dimension "d872" = 2
  dimension "d873" = 2
  dimension "d876" = 5
  dimension "d882" = 2
  dimension "d899" = 17
  dimension "d901" = 34
  dimension "d902" = 2
  dimension "d910" = 5
  dimension "d912" = 5
  dimension "d913" = 5
  dimension "d914" = 5
  dimension "d916" = 2
  dimension "d918" = 3
  dimension "d921" = 2.5
  dimension "d922" = 2.5
  dimension "d923" = 2.5
  dimension "d924" = 2.5
  dimension "d925" = 2
  dimension "d926" = 2
  constraint perpendicular L6 L7
  constraint tangent L6 A0
  constraint tangent L6 A1
  constraint tangent L7 A1
  constraint vertical L14
  constraint vertical L8
  constraint horizontal L9
  constraint tangent L8 A2
  constraint tangent L9 A2
  constraint tangent L7 A3
  constraint horizontal L10
  constraint horizontal L11
  constraint horizontal L12
  constraint vertical L13
  constraint coincident L12.start L14
  constraint collinear L14 L15
  constraint tangent L18 A4
  constraint tangent L19 A4
  constraint tangent L18 A5
  constraint equal A4 A5
  constraint horizontal L362
  constraint perpendicular L72 L362
  constraint tangent L72 A29
  constraint tangent L72 A30
  constraint tangent A30 L362
  constraint tangent A23 L362
  constraint horizontal L75
  constraint vertical L79
  constraint tangent L77 A27
  constraint tangent L73 A27
  constraint tangent A24 L77
  constraint equal A24 A27
  constraint vertical L129
  constraint vertical L123
  constraint horizontal L133
  constraint horizontal L122
  constraint vertical L104
  constraint tangent L123 A39
  constraint tangent L133 A39
  constraint horizontal L136
  constraint vertical L102
  constraint coincident L111.end L129
  constraint collinear L111 L129
  constraint tangent L110 A40
  constraint tangent L112 A40
  constraint tangent L107 A41
  constraint tangent L131 A41
  constraint equal A40 A41
  constraint concentric A42 A44
  constraint concentric A43 A45
  constraint tangent L137 A44
  constraint tangent L138 A44
  constraint tangent L139 A45
  constraint tangent L140 A45
  constraint tangent L137 A46
  constraint tangent L138 A47
  constraint equal A46 A47
  constraint tangent L139 A48
  constraint equal A46 A48
  constraint tangent L140 A49
  constraint equal A46 A49
  constraint coincident L46 L141.end
  constraint perpendicular L48 L141
  constraint tangent A28 L142
  constraint tangent A21 L143
  constraint tangent A29 L144
  constraint tangent L146 A56
  constraint tangent A56 L298
  constraint tangent L145 A57
  constraint tangent L146 A57
  constraint tangent L147 A58
  constraint tangent L148 A58
  constraint tangent L148 A59
  constraint tangent L147 A60
  constraint tangent L149 A61
  constraint tangent A61 L301
  constraint tangent A62 L301
  constraint tangent L150 A62
  constraint tangent L150 A76
  constraint tangent A76 L303
  constraint tangent A63 A78
  constraint tangent A63 L303
  constraint tangent A70 A73
  constraint tangent A73 A149
  constraint equal A64 A73
  constraint tangent A65 A70
  constraint equal A64 A65
  constraint tangent A66 A67
  constraint equal A64 A66
  constraint collinear L298 L299
  constraint coincident L213.end A73
  constraint concentric A73 A74
  constraint coincident L232 L300.start
  constraint coincident L297.end L301
  constraint collinear L301 L302
  constraint concentric A76 A77
  constraint collinear L303 L304
  constraint equal A88 A89
  constraint tangent A90 L670
  constraint tangent L323 A91
  constraint tangent L324 A91
  constraint tangent A47 L325
  constraint horizontal L325
  constraint tangent A48 L326
  constraint tangent A49 L327
  constraint perpendicular L326 L327
  constraint tangent A46 L328
  constraint tangent L325 A94
  constraint tangent L326 A94
  constraint tangent L327 A95
  constraint tangent L328 A95
  constraint equal A94 A95
  constraint tangent A89 L666
  constraint tangent A89 L668
  constraint tangent A96 L668
  constraint tangent A96 L331
  constraint vertical L329
  constraint tangent A97 L332
  constraint tangent L329 A98
  constraint tangent A98 L666
  constraint tangent L329 A99
  constraint tangent L331 A99
  constraint equal A98 A99
  constraint tangent L330 A100
  constraint equal A98 A100
  constraint tangent L330 A101
  constraint equal A98 A101
  constraint perpendicular L109 L333
  constraint perpendicular L134 L334
  constraint concentric A102 A105
  constraint concentric A103 A104
  constraint tangent L335 A104
  constraint vertical L335
  constraint perpendicular L335 L336
  constraint perpendicular L336 L337
  constraint tangent L339 A105
  constraint perpendicular L336 L339
  constraint perpendicular L339 L340
  constraint tangent L335 A106
  constraint tangent L336 A106
  constraint tangent L339 A107
  constraint tangent L340 A107
  constraint equal A106 A107
  constraint tangent L336 A108
  constraint tangent L337 A108
  constraint tangent L338 A109
  constraint tangent L340 A109
  constraint equal A108 A109
  constraint tangent L339 A110
  constraint tangent A105 A110
  constraint tangent L335 A111
  constraint tangent A104 A111
  constraint equal A110 A111
  constraint tangent L337 A112
  constraint tangent A105 A112
  constraint tangent L338 A113
  constraint tangent A104 A113
  constraint equal A112 A113
  constraint horizontal L341
  constraint vertical L342
  constraint horizontal L343
  constraint vertical L344
  constraint horizontal L345
  constraint vertical L346
  constraint horizontal L347
  constraint vertical L348
  constraint perpendicular L11 L349
  constraint perpendicular L90 L350
  constraint collinear L352 L353
  constraint tangent L352 A114
  constraint tangent L353 A115
  constraint tangent L351 A116
  constraint tangent L351 A117
  constraint perpendicular L354 L357
  constraint perpendicular L354 L355
  constraint perpendicular L356 L357
  constraint collinear L357 L358
  constraint tangent L356 A118
  constraint tangent L357 A118
  constraint tangent L354 A119
  constraint tangent L358 A119
  constraint equal A118 A119
  constraint tangent L355 A120
  constraint tangent L356 A120
  constraint tangent L354 A121
  constraint tangent L355 A121
  constraint equal A120 A121
  constraint collinear L362 L363
  constraint concentric A50 A130
  constraint parallel L366 L367
  constraint tangent L366 A131
  constraint tangent L366 A132
  constraint tangent A130 A132
  constraint tangent L367 A133
  constraint tangent A130 A133
  constraint equal A132 A133
  constraint tangent L367 A134
  constraint equal A132 A134
  constraint concentric A51 A139
  constraint tangent A134 A139
  constraint concentric A85 A140
  constraint tangent A138 A140
  constraint perpendicular L370 L805
  constraint perpendicular L371 L805
  constraint tangent L370 A141
  constraint tangent A139 A141
  constraint tangent A142 L805
  constraint tangent L370 A142
  constraint equal A141 A142
  constraint tangent L371 A143
  constraint tangent A140 A143
  constraint equal A141 A143
  constraint tangent A144 L805
  constraint tangent L371 A144
  constraint equal A141 A144
  constraint vertical L373
  constraint vertical L375
  constraint tangent L373 A145
  constraint tangent L375 A146
  constraint tangent L375 A147
  constraint tangent L373 A148
  constraint concentric A149 A150
  constraint perpendicular L214 L561
  constraint perpendicular L522 L562
  constraint tangent L167 A177
  constraint tangent A150 A177
  constraint tangent A11 L563
  constraint tangent A16 L564
  constraint perpendicular L315 L566
  constraint horizontal L568
  constraint vertical L569
  constraint horizontal L570
  constraint vertical L571
  constraint perpendicular L577 L578
  constraint perpendicular L580 L581
  constraint tangent L580 A180
  constraint tangent L578 A181
  constraint tangent A90 L583
  constraint tangent A36 L584
  constraint perpendicular L114 L585
  constraint coincident A185.centre L598.start
  constraint perpendicular L598 L613
  constraint coincident A184.centre L597.start
  constraint perpendicular L597 L613
  constraint tangent A33 L604
  constraint perpendicular L99 L605
  constraint tangent A31 L607
  constraint vertical L607
  constraint perpendicular L609 L613
  constraint perpendicular L609 L610
  constraint collinear L613 L614
  constraint perpendicular L624 L625
  constraint collinear L628 L629
  constraint perpendicular L580 L639
  constraint perpendicular L581 L640
  constraint perpendicular L580 L641
  constraint perpendicular L581 L642
  constraint perpendicular L645 L646
  constraint perpendicular L646 L647
  constraint perpendicular L647 L648
  constraint vertical L649
  constraint tangent L645 A190
  constraint coincident P13 L646
  constraint coincident P13 L647
  constraint tangent L646 A191
  constraint tangent L647 A191
  constraint coincident P14 L647
  constraint coincident P14 L648
  constraint tangent L647 A192
  constraint tangent L648 A192
  constraint equal A191 A192
  constraint tangent L648 A193
  constraint tangent L649 A193
  constraint equal A191 A193
  constraint concentric A195 A196
  constraint equal A197 A198
  constraint tangent A196 A199
  constraint equal A197 A199
  constraint tangent A196 A200
  constraint equal A197 A200
  constraint tangent L649 A201
  constraint tangent A190 A201
  constraint tangent A206 L658
  constraint parallel L657 L658
  constraint perpendicular L657 L659
  constraint tangent L658 A209
  constraint tangent L659 A209
  constraint tangent L657 A210
  constraint tangent L659 A210
  constraint equal A209 A210
  constraint tangent A100 L660
  constraint tangent A101 L661
  constraint horizontal L662
  constraint vertical L663
  constraint horizontal L664
  constraint vertical L665
  constraint tangent L662 A211
  constraint tangent L663 A211
  constraint tangent L662 A212
  constraint tangent L665 A212
  constraint equal A211 A212
  constraint tangent L664 A213
  constraint tangent L665 A213
  constraint equal A211 A213
  constraint tangent L663 A214
  constraint tangent L664 A214
  constraint equal A211 A214
  constraint concentric A86 A222
  constraint concentric A87 A215
  constraint collinear L666 L667
  constraint concentric A215 A216
  constraint collinear L668 L669
  constraint collinear L670 L671
  constraint concentric A222 A223
  constraint tangent L667 A224
  constraint tangent A222 A224
  constraint tangent L672 A225
  constraint tangent A223 A225
  constraint equal A224 A225
  constraint tangent L677 A226
  constraint tangent A223 A226
  constraint equal A224 A226
  constraint tangent L666 A227
  constraint tangent A222 A227
  constraint equal A224 A227
  constraint tangent A220 A228
  constraint tangent L676 A228
  constraint equal A224 A228
  constraint tangent L675 A229
  constraint tangent A220 A229
  constraint equal A224 A229
  constraint tangent A215 A230
  constraint tangent L668 A230
  constraint equal A224 A230
  constraint tangent A215 A231
  constraint tangent L669 A231
  constraint equal A224 A231
  constraint tangent A216 A232
  constraint tangent L670 A232
  constraint equal A224 A232
  constraint tangent A216 A233
  constraint tangent L671 A233
  constraint equal A224 A233
  constraint tangent A178 A243
  constraint tangent A240 A243
  constraint tangent A179 A244
  constraint tangent A241 A244
  constraint concentric A242 A245
  constraint concentric A245 A246
  constraint tangent A240 A247
  constraint tangent A246 A247
  constraint tangent A241 A248
  constraint tangent A246 A248
  constraint equal A247 A248
  constraint tangent A202 L683
  constraint tangent A203 L684
  constraint collinear L685 L686
  constraint tangent L683 A249
  constraint tangent L685 A249
  constraint tangent L684 A250
  constraint tangent L686 A250
  constraint equal A249 A250
  constraint collinear L687 L688
  constraint tangent L688 A251
  constraint tangent L687 A252
  constraint equal A251 A252
  constraint perpendicular L685 L722
  constraint tangent A296 L912
  constraint parallel L318 L756
  constraint parallel L319 L759
  constraint tangent L758 A302
  constraint tangent L757 A302
  constraint tangent L757 A303
  constraint tangent A303 L759
  constraint equal A302 A303
  constraint tangent A304 L759
  constraint tangent L756 A304
  constraint equal A302 A304
  constraint tangent L756 A305
  constraint equal A302 A305
  constraint coincident L485 L758.end
  constraint coincident L448 L456.end
  constraint collinear L759 L760
  constraint coincident A304 L456.start
  constraint coincident L385.end A305
  constraint concentric A305 A306
  constraint horizontal L796
  constraint horizontal L797
  constraint vertical L798
  constraint horizontal L799
  constraint vertical L800
  constraint tangent L797 A319
  constraint tangent L800 A319
  constraint tangent L799 A320
  constraint tangent L800 A320
  constraint equal A319 A320
  constraint tangent L798 A321
  constraint tangent L799 A321
  constraint equal A319 A321
  constraint tangent L797 A322
  constraint tangent L798 A322
  constraint equal A319 A322
  constraint concentric A292 A327
  constraint collinear L805 L806
  constraint collinear L806 L807
  constraint collinear L807 L808
  constraint tangent A327 A330
  constraint tangent L805 A330
  constraint tangent A327 A331
  constraint tangent L806 A331
  constraint equal A330 A331
  constraint tangent L806 A332
  constraint tangent A328 A332
  constraint equal A330 A332
  constraint tangent A328 A333
  constraint tangent L807 A333
  constraint equal A330 A333
  constraint tangent L807 A334
  constraint tangent A329 A334
  constraint equal A330 A334
  constraint tangent L808 A335
  constraint tangent A329 A335
  constraint equal A330 A335
  constraint coincident L528.end L809
  constraint collinear L809 L810
  constraint tangent A336 L811
  constraint tangent A337 L812
  constraint tangent L811 A337
  constraint tangent L812 A338
  constraint tangent L813 A340
  constraint tangent L813 A339
  constraint tangent A198 L840
  constraint tangent A369 L841
  constraint tangent A200 L842
  constraint tangent A371 L843
  constraint tangent A7 L844
  constraint tangent A20 L845
  constraint tangent A0 L846
  constraint tangent A15 L847
  constraint tangent A5 L848
  constraint tangent A8 L849
  constraint tangent A338 L851
  constraint parallel L850 L851
  constraint perpendicular L850 L852
  constraint tangent A336 L853
  constraint tangent L851 A375
  constraint tangent L852 A375
  constraint tangent L850 A376
  constraint tangent L852 A376
  constraint equal A375 A376
  constraint tangent L850 A377
  constraint tangent L853 A377
  constraint equal A375 A377
  constraint perpendicular L119 L872
  constraint parallel L872 L878
  constraint tangent A396 A400
  constraint tangent L878 A396
  constraint tangent A397 A400
  constraint tangent L878 A397
  constraint equal A396 A397
  constraint horizontal L879
  constraint horizontal L880
  constraint coincident A10.centre L880.start
  constraint vertical L881
  constraint vertical L882
  constraint concentric A398 A399
  constraint concentric A400 A401
  constraint tangent A399 A402
  constraint tangent A401 A402
  constraint tangent A399 A403
  constraint tangent A400 A403
  constraint equal A402 A403
  constraint concentric A411 A412
  constraint tangent A412 A413
  constraint tangent A315 A413
  constraint tangent A314 A414
  constraint tangent A412 A414
  constraint equal A413 A414
  constraint perpendicular L143 L896
  constraint perpendicular L896 L897
  constraint parallel L896 L898
  constraint tangent L896 A423
  constraint tangent L897 A423
  constraint tangent L897 A424
  constraint tangent L898 A424
  constraint equal A423 A424
  constraint tangent A339 L900
  constraint tangent A421 L901
  constraint perpendicular L814 L909
  constraint perpendicular L142 L910
  constraint perpendicular L910 L911
  constraint tangent L909 A431
  constraint tangent L911 A431
  constraint tangent L910 A432
  constraint tangent L911 A432
  constraint equal A431 A432
  constraint concentric A295 A433
  constraint tangent A433 A434
  constraint tangent L912 A434
  constraint tangent A433 A435
  constraint tangent A296 A435
  constraint tangent A255 L913
  constraint tangent A128 L915
  constraint tangent A256 L916
  constraint tangent A265 L917
  constraint tangent A264 L919
  constraint tangent A346 L921
  constraint tangent A272 L922
  constraint tangent A275 L923
  constraint tangent A114 L925
  constraint tangent A251 L926
  constraint tangent A252 L927
  constraint tangent A115 L928
  constraint horizontal L932
  constraint vertical L933
  constraint horizontal L930
  constraint vertical L929
  constraint concentric A436 A441
  constraint concentric A438 A440
  constraint concentric A439 A443
  constraint concentric A437 A442
  constraint coincident A438 L931.start
  constraint collinear L930 L931
  constraint tangent L929 A444
  constraint tangent A441 A444
  constraint tangent A441 A445
  constraint tangent L932 A445
  constraint equal A444 A445
  constraint tangent L929 A446
  constraint tangent A440 A446
  constraint equal A444 A446
  constraint tangent L930 A447
  constraint tangent A440 A447
  constraint equal A444 A447
  constraint tangent L930 A448
  constraint tangent A443 A448
  constraint equal A444 A448
  constraint tangent L933 A449
  constraint tangent A443 A449
  constraint equal A444 A449
  constraint tangent A442 A450
  constraint tangent L933 A450
  constraint equal A444 A450
  constraint tangent A442 A451
  constraint tangent L932 A451
  constraint equal A444 A451
  constraint concentric A452 A454
  constraint tangent L934 A455
  constraint tangent A454 A456
  constraint tangent L935 A456
  constraint equal A455 A456
  constraint tangent A454 A457
  constraint tangent L934 A457
  constraint equal A455 A457
  constraint tangent L936 A459
  constraint tangent L937 A459
  constraint parallel L936 L937
  constraint perpendicular L342 L938
  constraint perpendicular L938 L939
  constraint perpendicular L939 L940
  constraint perpendicular L938 L941
  constraint horizontal L946
  constraint coincident P15 L938
  constraint coincident P15 L939
  constraint tangent L938 A462
  constraint tangent L939 A462
  constraint tangent L941 A463
  constraint tangent L942 A463